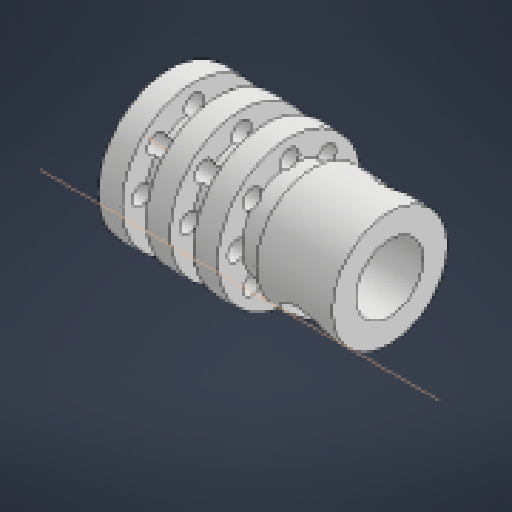
# Autodesk Inventor part: felga
Saved by Autodesk Inventor 2023 (Build 270158000, 158)
## iProperties
Created: 2024-02-27
Part Number: felga
Material: Generic
Document SubType Name: Modeling
Designer: Michał
Density: 1 g/cm^3
Appearance: Default
Author: Michał
Autodesk Inventor part; units mm, degrees
ref_plane "YZ Plane" through (0, 0, 0) normal (1, 0, 0) x (0, 1, 0)
ref_plane "XZ Plane" through (0, 0, 0) normal (0, 1, 0) x (-1, 0, 0)
ref_plane "XY Plane" through (0, 0, 0) normal (0, 0, 1) x (1, 0, 0)
sketch "Sketch1" plane through (0, 0, 0) normal (0, 1, 0) x (-1, 0, 0)
  line L0 (0, 0) -> (23, 0)
  line L1 (23, 0) -> (23, 5)
  line L2 (0, 0) -> (0, 6)
  line L3 (0, 6) -> (8, 6)
  line L4 (8, 6) -> (8, 5)
  line L5 (8, 5) -> (10.5, 5)
  line L6 (10.5, 5) -> (10.5, 7.5)
  line L7 (10.5, 7.5) -> (13, 7.5)
  line L8 (13, 7.5) -> (13, 5)
  line L9 (13, 5) -> (15.5, 5)
  line L10 (15.5, 5) -> (15.5, 7.5)
  line L11 (15.5, 7.5) -> (18, 7.5)
  line L12 (18, 7.5) -> (18, 5)
  line L13 (18, 5) -> (20.5, 5)
  line L14 (20.5, 5) -> (20.5, 7.5)
  line L15 (20.5, 7.5) -> (23, 7.5)
  line L16 (23, 7.5) -> (23, 5)
  line L17 (0, 3.5) -> (15, 3.5)
  line L18 (15, 3.5) -> (15, 0)
  point P0 (19.25, 5)
  dimension "d0" = 2.5
  dimension "d1" = 2.5
  dimension "d4" = 5
  dimension "d9" = 8
  dimension "d10" = 6
  dimension "d11" = 7.5
  dimension "d12" = 2.5
  dimension "d13" = 3.5
  dimension "d14" = 15
  constraints: 38 end point, 8 perpendicular, 5 point on line, 3 horizontal, 1 coincident, 1 midpoint, 1 vertical, 18 other
  measures "d0" distance of L4.end L5.end
  measures "d1" distance of L6.end L7.end
  measures "d4" distance of L4.end L9.start
  measures "d9" distance between parallel lines of L4 L2
  measures "d10" distance between parallel lines of L0 L3
  measures "d11" distance between parallel lines of L0 L15
  measures "d12" distance from line of L15 point (19.25, 5)
  measures "d13" distance between parallel lines of L0 L17
  measures "d14" distance between parallel lines of L2 L18
revolve "Revolution1" add sketch "Sketch1" angle 360 about axis through (0, 0, 0) along (-1, 0, 0) contours L18 L17 L2 L3 L4 L5 L6 L7 L8 L9 L10 L11 L12 L13 L14 L15 L16 L1 L0
sketch "Sketch2" plane through (-23, 0, 0) normal (-1, 0, 0) x (0, 0, 1)
  circle A0 centre (0, 0) radius 5.5 construction
  circle A1 centre (0, 0) radius 7.5 construction
  point P0 (-5.5, 0)
  point P1 (-3.8891, -3.8891)
  point P2 (0, -5.5)
  point P3 (3.8891, -3.8891)
  point P4 (5.5, 0)
  point P5 (3.8891, 3.8891)
  point P6 (0, 5.5)
  point P7 (-3.8891, 3.8891)
  dimension "d16" = 2
  dimension "d19" = 360
  constraints: 2 horizontal alignment, 1 coincident, 11 other
hole "Hole1" at (-23, 0, -5.5) at (-23, -3.8891, -3.8891) at (-23, -5.5, 0) at (-23, -3.8891, 3.8891) at (-23, 0, 5.5) at (-23, 3.8891, 3.8891) at (-23, 5.5, 0) at (-23, 3.8891, -3.8891) direction (1, 0, 0) diameter 2 depth 12.5 tip angle 118
ref_plane "Work Plane4" through (-4, -4.2426, 4.2426) normal (0, 0.7071068, -0.7071068) x (0, 0.7071068, 0.7071068)
ref_plane "Work Plane3" through (-20.5, -4.5962, -4.5962) normal (0, 0.7071068, -0.7071068) x (0, 0.7071068, 0.7071068)
sketch "Sketch4" plane through (-4, -4.2426, 4.2426) normal (0, 0.7071068, -0.7071068) x (0, 0.7071068, 0.7071068)
  line L0 (-6, -4) -> (6, -4) construction
  line L1 (0, -4) -> (0, 4) construction
  point P0 (0, 0)
  constraints: 2 end point, 2 midpoint, 1 vertical
hole "Hole3" at (-4, -4.2426, 4.2426) direction (0, 0.7071068, -0.7071068) diameter 3.4 end through all counterbore diameter 5.7 counterbore depth 2 clearance for "Hex Head Cap Screw ISO 24017" size "M3" standard "ISO"
equation "\"d4\" = d0 + d1"
body "Solid1"
